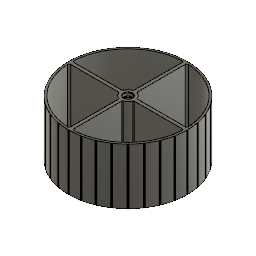
textureWheel2 (Autodesk Fusion 360 design; units mm, degrees)
Autodesk Fusion 360 part; units mm, degrees
note: some values were not read from the file. Chosen so that the rebuilt part matches the saved one: which face or edge a step refers to; that a step has no effect. Set by a fixed rule: which sketch regions a step uses.
mesh "Mesh1" [no effect]
sketch "Sketch2" plane through (0, 0, 0) normal (0, 1, 0) x (1, 0, 0)
  circle A0 centre (0, 0) radius 73
  line L0 (2, 71) -> (-2, 71)
  line L1 (-2, 71) -> (-2, -71)
  line L2 (-2, -71) -> (2, -71)
  line L3 (2, -71) -> (2, 71)
  line L4 (2, 71) -> (-2, -71) construction
  line L5 (-2, 71) -> (2, -71) construction
  line L6 (-71, 2) -> (71, 2)
  line L7 (71, 2) -> (71, -2)
  line L8 (71, -2) -> (-71, -2)
  line L9 (-71, -2) -> (-71, 2)
  line L10 (-71, 2) -> (71, -2) construction
  line L11 (71, 2) -> (-71, -2) construction
  circle A1 centre (0, 0) radius 9
  circle A2 centre (0, 0) radius 70.5
  dimension "d3" = 146
  dimension "d5" = 142
  dimension "d6" = 4
  dimension "d7" = 142
  dimension "d8" = 4
  dimension "d9" = 18
  dimension "d11" = 141
  measures "d3" diameter of A0
  measures "d9" diameter of A1
  measures "d11" diameter of A2
extrude "Extrude1" add sketch "Sketch2" along normal blind 69 contours A0 | L0 L1 L3 A2 | L1 L3 A1 A2 | L3 L6 A1 | L1 L3 L6 A1 | L6 L8 A1 A2 | L6 L7 L8 A2 | L1 L6 A1 | L6 L8 L9 A2 | L6 L8 A1 A2 | L3 L6 L8 A1 | L1 L3 L6 L8 | L1 L6 L8 A1 | L3 L8 A1 | L1 L3 L8 A1 | L1 L8 A1 | L1 L2 L3 A2 | L1 L3 A1 A2
sketch "Sketch3" plane through (0, 69, 0) normal (0, 1, 0) x (-1, 0, 0)
  line L0 (8.775, -2) -> (70.4716, -2)
  arc A0 (2, -70.4716) -> (70.4716, -2) centre (0, 0) ccw
  line L1 (2, -70.4716) -> (2, -8.775)
  arc A1 (2, -8.775) -> (8.775, -2) centre (0, 0) ccw
  arc A2 (70.4716, 2) -> (2, 70.4716) centre (0, 0) ccw
  line L2 (70.4716, 2) -> (8.775, 2)
  arc A3 (8.775, 2) -> (2, 8.775) centre (0, 0) ccw
  line L3 (2, 8.775) -> (2, 70.4716)
  arc A4 (-2, 70.4716) -> (-70.4716, 2) centre (0, 0) ccw
  line L4 (-2, 70.4716) -> (-2, 8.775)
  arc A5 (-2, 8.775) -> (-8.775, 2) centre (0, 0) ccw
  line L5 (-8.775, 2) -> (-70.4716, 2)
  arc A6 (-8.775, -2) -> (-2, -8.775) centre (0, 0) ccw
  line L6 (-2, -8.775) -> (-2, -70.4716)
  arc A7 (-70.4716, -2) -> (-2, -70.4716) centre (0, 0) ccw
  line L7 (-70.4716, -2) -> (-8.775, -2)
  circle A8 centre (0, 0) radius 73
  circle A9 centre (0, 72.5) radius 0.7
  dimension "d14" = 1.4
  measures "d14" diameter of A9
extrude "Extrude2" add sketch "Sketch3" against normal blind 69 contours A8 A9 | A8 A9 picked at (-0.0074, 72.6) picked at (0.0165, 73.066)
fillet "Fillet1" radius 1 1 edges at (0.4916, 34.5, 72.9983)
fillet "Fillet2" radius 1 1 edges at (-0.4916, 34.5, 72.9983)
pattern_circular "C-Pattern1" count 32 over 360 about axis through (0, 0, 0) along (0, 1, 0) of 3 faces at (0.637, 23, 73.0104) (0.1903, 23, 73.1737) (-0.7171, 23, 72.9997)
hole "Hole1" at (0, 69, 0) direction (0, -1, 0) diameter 8.1 depth 69 tip angle 180
hole "Hole2" at (0, 69, 0) direction (0, -1, 0) diameter 10.1 depth 4 tip angle 180
fillet "Fillet3" radius 0.6 1 edges at (-1.4645, 65, -3.7759)
fillet "Fillet4" radius 0.6 1 edges at (1.8262, 69, -4.7083)
fillet "Fillet5" radius 2 8 edges at (-2, 34.5, 70.4716) (70.4716, 34.5, -2) (70.4716, 34.5, 2) (2, 34.5, -70.4716) (-70.4716, 34.5, -2) (-70.4716, 34.5, 2) (-2, 34.5, -70.4716) (2, 34.5, 70.4716)
fillet "Fillet6" radius 1 2 edges at (8.775, 34.5, -2) (2, 34.5, -8.775)
fillet "Fillet7" radius 1 6 edges at (-2, 34.5, -8.775) (-8.775, 34.5, -2) (-8.775, 34.5, 2) (-2, 34.5, 8.775) (2, 34.5, 8.775) (8.775, 34.5, 2)
fillet "Fillet8" radius 0.6 1 edges at (-1.4645, 0, -3.7759)
